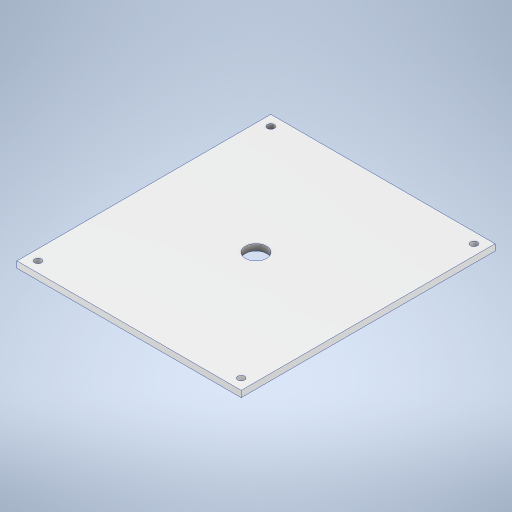
# Autodesk Inventor part: link2_plate3
Saved by Autodesk Inventor 2024 (Build 280153000, 153)
## iProperties
Created: 2024-12-13
Part Number: link2_plate3
Material: アルミニウム 6061
Document SubType Name: Sheet Metal
Designer: hirek
Density: 2.7 g/cm^3
Sheet Metal Rule: Default_mm
Appearance: アルミニウム - フラット
Author: hirek
Autodesk Inventor part; units mm, degrees
ref_plane "YZ Plane" through (0, 0, 0) normal (1, 0, 0) x (0, 1, 0)
ref_plane "XZ Plane" through (0, 0, 0) normal (0, 1, 0) x (-1, 0, 0)
ref_plane "XY Plane" through (0, 0, 0) normal (0, 0, 1) x (1, 0, 0)
sketch "スケッチ1" plane through (0, 0, 0) normal (0, 1, 0) x (-1, 0, 0)
  line L0 (0, 0) -> (106, 0)
  line L1 (106, 0) -> (106, -120)
  line L2 (106, -120) -> (0, -120)
  line L3 (0, -120) -> (0, 0)
  dimension "d0" = 106
  dimension "d1" = 120
  constraints: 8 end point, 2 parallel, 1 horizontal, 1 perpendicular
  measures "d0" distance of L1.end L2.end
  measures "d1" distance of L0.end L1.end
extrude "押し出し1" add sketch "スケッチ1" along normal blind 3
sketch "スケッチ4" plane through (0, 3, 0) normal (0, 1, 0) x (1, 0, 0)
  line L0 (-106, 120) -> (-106, 0) projected
  line L1 (-106, 5) -> (0, 5)
  line L2 (0, 0) -> (0, 120) projected
  line L3 (-120, 115) -> (0, 115)
  line L4 (-106, 0) -> (0, 0) projected
  line L5 (0, 120) -> (-106, 120) projected
  line L6 (-106, 0) -> (0, 0) projected
  line L7 (-101, 0) -> (-101, 120)
  line L8 (-5, 120) -> (-5, 0)
  point P0 (-101, 5)
  point P1 (-5, 5)
  point P2 (-5, 115)
  point P3 (-101, 115)
  dimension "d22" = 5
  dimension "d23" = 5
  dimension "d24" = 5
  dimension "d25" = 5
  constraints: 14 point on line, 8 end point, 2 horizontal, 2 perpendicular
  measures "d22" distance between parallel lines of L1 L4
  measures "d23" distance between parallel lines of L5 L3
  measures "d24" distance between parallel lines of L0 L7
  measures "d25" distance between parallel lines of L2 L8
hole "穴2" at (-101, 3, -5) at (-5, 3, -5) at (-5, 3, -115) at (-101, 3, -115) direction (0, -1, 0) diameter 3.2 end through all
sketch "スケッチ5" plane through (0, 3, 0) normal (0, 1, 0) x (1, 0, 0)
  line L0 (-106, 120) -> (-106, 0) projected
  line L1 (-106, 60) -> (0, 60)
  line L2 (0, 0) -> (0, 120) projected
  point P0 (-53, 60)
  constraints: 3 midpoint, 2 end point
hole "穴3" at (-53, 3, -60) direction (0, -1, 0) diameter 10 end through all
equation "\"d38\" = Thickness"
equation "\"BendRadius\" = Thickness"
equation "\"BendReliefWidth\" = Thickness"
equation "\"BendReliefDepth\" = 0.5 * Thickness"
equation "\"CornerReliefSize\" = 4 * Thickness"
equation "\"MinimumRemnant\" = 2 * Thickness"
equation "\"TransitionRadius\" = BendRadius"
equation "\"JacobiRadiusSize\" = BendRadius"
equation "\"GapSize\" = Thickness"
equation "\"Thickness\" = 0.5"
